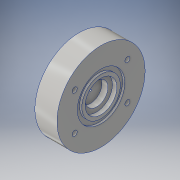
# Autodesk Inventor part: .5 in hole
Saved by Autodesk Inventor 2016 (Build 200138000, 138)
## iProperties
Created: 2016-06-27
Part Number: .5 in hole
Material: Aluminum 6061
Document SubType Name: Modeling
Designer: Jonathan
Density: 2.7 g/cm^3
Appearance: Aluminum - Flat
Author: Jonathan
Autodesk Inventor part; units mm, degrees
ref_plane "YZ Plane" through (0, 0, 0) normal (1, 0, 0) x (0, 1, 0)
sketch "Sketch1" plane through (0, 0, 0) normal (1, 0, 0) x (0, 1, 0)
  circle A0 centre (0, 0) radius 25.4
  dimension "d0" = 50.8
  constraints: 1 centre point, 1 coincident
  measures "d0" diameter of A0
extrude "Extrusion1" add sketch "Sketch1" along normal blind 12.7
sketch "Sketch10" plane through (12.7, 0, 0) normal (1, 0, 0) x (0, 0, -1)
  point P0 (0, 0)
  point P1 (0, 0)
  constraints: 1 coincident
hole "Hole4" at (12.7, 0, 0) direction (-1, 0, 0) diameter 18.2563 depth 2.54
ref_plane "Work Plane2" through (11.43, 0, 0) normal (1, 0, 0) x (0, 0, -1)
hole "Hole1" at (11.43, 0, 0) direction (-1, 0, 0) diameter 13.0969 depth 4.7625
ref_plane "Work Plane1" through (-12.7, 0, 0) normal (1, 0, 0) x (0, 0, -1)
sketch "Sketch5" plane through (0, 0, 0) normal (1, 0, 0) x (0, 1, 0)
  line L0 (0, 9) -> (0, -9)
  circle A0 centre (0, 0) radius 25.4 projected
  line L1 (-15.24, 0) -> (15.24, 0)
  line L2 (-15.24, 10.795) -> (-15.24, -10.795)
  dimension "d37" = 18
  dimension "d45" = 30.48
  dimension "d46" = 21.59
  constraints: 6 end point, 4 coincident, 3 midpoint, 2 vertical, 1 parallel, 1 perpendicular
  measures "d37" distance of L0.start L0.end
  measures "d45" distance of L1.start L1.end
  measures "d46" distance of L2.start L2.end
hole "Hole2" at (0, 0, -9) direction (1, 0, 0) diameter 2.159 depth 8.8646 tip angle 118
sketch "Sketch6" plane through (0, 0, 0) normal (-1, 0, 0) x (0, 0, 1)
  circle A0 centre (0, 0) radius 0.5715
  dimension "d34" = 1.143
  constraints: 1 centre point, 1 coincident
  measures "d34" diameter of A0
hole "Hole5" at (0, 0, 0) direction (1, 0, 0) diameter 1 end through all
mirror "Mirror1" about plane through (0, 0, 0) normal (0, 0, 1) of "Hole2"
hole "Hole3" at (0, -15.24, 10.795) at (0, -15.24, -10.795) direction (1, 0, 0) diameter 2.9464 end through all counterbore diameter 4.826 counterbore depth 3.302 clearance for "Socket Head Cap Screw" size "#4" standard "Ansi Unified Screw Threads"
mirror "Mirror2" about plane through (0, 0, 0) normal (0, 1, 0) of "Hole3"
sketch "Sketch9" plane through (0, 0, 0) normal (0, 1, 0) x (-1, 0, 0)
  line L0 (-11.4554, -11.1125) -> (-12.7, -11.1125)
  line L1 (-12.7, -11.1125) -> (-12.7, -13.6525)
  line L2 (-12.7, -13.6525) -> (-11.4554, -13.6525)
  line L3 (-11.4554, -13.6525) -> (-11.4554, -11.1125)
  line L4 (2.54, 0) -> (-15.24, 0) projected
  line L5 (-12.7, 25.4) -> (-12.7, -25.4) projected
  point P0 (0, 0)
  dimension "d55" = 2.54
  dimension "d56" = 1.2446
  dimension "d59" = 11.1125
  constraints: 8 end point, 2 parallel, 1 collinear, 1 perpendicular
  measures "d55" distance of L2.end L0.start
  measures "d56" distance of L1.end L2.end
  measures "d59" distance between parallel lines of L4 L0
revolve "Revolution1" cut sketch "Sketch9" angle 360 about axis through (-10, 0, 0) along (1, 0, 0)
body "Solid1"
